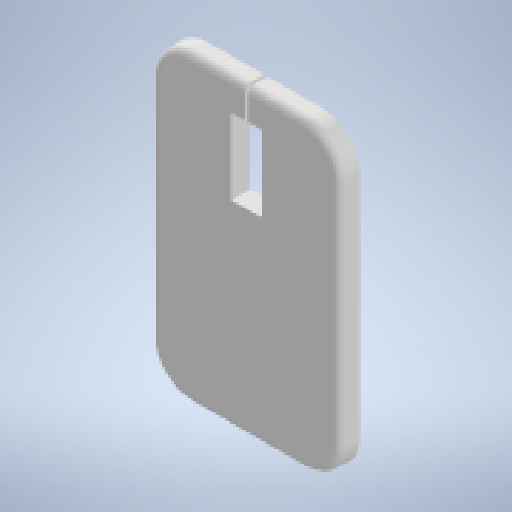
# Autodesk Inventor part: Tampa
Saved by Autodesk Inventor 2025 (Build 290162010, 162A)
## iProperties
Created: 2025-10-21
Part Number: Tampa
Material: Genérico
Document SubType Name: Modeling
Designer: 202321250026
Density: 1 g/cm^3
Appearance: Padrão
Author: 202321250026
Autodesk Inventor part; units mm, degrees
ref_plane "YZ Plane" through (0, 0, 0) normal (1, 0, 0) x (0, 1, 0)
ref_plane "XZ Plane" through (0, 0, 0) normal (0, 1, 0) x (-1, 0, 0)
ref_plane "XY Plane" through (0, 0, 0) normal (0, 0, 1) x (1, 0, 0)
sketch "Esboço3" plane through (0, 0, 0) normal (0, 0, 1) x (1, 0, 0)
  arc A0 (-23, -30) -> (-15, -38) centre (-15, -30) ccw projected
  line L0 (-23, -30) -> (-23, 30) projected
  arc A1 (-15, 38) -> (-23, 30) centre (-15, 30) ccw projected
  line L1 (-15, 38) -> (15, 38) projected
  arc A2 (23, 30) -> (15, 38) centre (15, 30) ccw projected
  line L2 (23, 30) -> (23, -30) projected
  arc A3 (15, -38) -> (23, -30) centre (15, -30) ccw projected
  line L3 (15, -38) -> (-15, -38) projected
  arc A4 (-25, -30) -> (-15, -40) centre (-15, -30) ccw projected
  line L4 (-15, -40) -> (15, -40) projected
  arc A5 (15, -40) -> (25, -30) centre (15, -30) ccw projected
  line L5 (25, -30) -> (25, 30) projected
  arc A6 (25, 30) -> (15, 40) centre (15, 30) ccw projected
  line L6 (15, 40) -> (-15, 40) projected
  arc A7 (-15, 40) -> (-25, 30) centre (-15, 30) ccw projected
  line L7 (-25, 30) -> (-25, -30) projected
  line L8 (-4, 12) -> (-4, 32) projected
  line L9 (-4, 32) -> (4, 32) projected
  line L10 (4, 12) -> (4, 32) projected
  line L11 (4, 12) -> (-4, 12) projected
  line L12 (-0.5, 40) -> (0.5, 40)
  line L13 (0.5, 40) -> (0.5, 32)
  line L14 (0.5, 32) -> (-0.5, 32)
  line L15 (-0.5, 32) -> (-0.5, 40)
  point P0 (0, 0)
  point P1 (0.5, 36)
  point P2 (0, 32)
  point P3 (-0.5, 38)
  point P4 (0.5, 38)
  dimension "d2" = 1
  dimension "d3" = 0
  dimension "d4" = 3.5
  constraints: 8 end point, 2 midpoint, 2 parallel, 1 horizontal, 1 perpendicular, 1 point on line
  measures "d2" distance from line of point (0.5, 36) L15
  measures "d3" distance from line of L9 point (0, 32)
  measures "d4" distance from line of L9.end L13
extrude "Extrusão1" add sketch "Esboço3" along normal blind 5 contours L0 A1 L1 L15 L9 L8 L11 L10 L13 A2 L2 A3 L3 A0 | A0 L3 A3 L2 A2 L1 L13 L6 A6 L5 A5 L4 A4 L7 A7 L15 A1 L0
fillet "Arredondamento1" radius 2 9 edges at (-22.0711, 37.0711, 5) (-25, 0, 5) (-22.0711, -37.0711, 5) (0, -40, 5) (22.0711, -37.0711, 5) (25, 0, 5) (22.0711, 37.0711, 5) (7.75, 40, 5) (-7.75, 40, 5)
shell "Casca1" thickness 2 removed faces 1 at (1.3333, -22.6667, 0)
